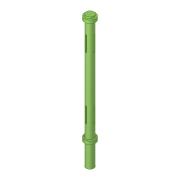
# Autodesk Inventor part: middleRod
Saved by Autodesk Inventor 2018 (Build 220112000, 112)
## iProperties
Created: 2017-11-16
Part Number: middleRod
Material: Aluminum 6061
Document SubType Name: Modeling
Designer: Udara Wanasinghe
Density: 2.7 g/cm^3
Appearance: Aluminum - Flat(1)
Mass: 41.1366 g
Surface Area: 69.3276 cm^2
Volume: 15.2358 cm^3
Author: Udara Wanasinghe
Autodesk Inventor part; units mm, degrees
ref_plane "XZ Plane" through (0, 0, 0) normal (0, 1, 0) x (-1, 0, 0)
ref_plane "XY Plane" through (0, 0, 0) normal (0, 0, 1) x (1, 0, 0)
sketch "Sketch1" plane through (0, 0, 0) normal (0, 1, 0) x (-1, 0, 0)
  circle A0 centre (0, 0) radius 5
  point P0 (0, 5)
  dimension "d0" = 10
  constraints: 1 coincident, 1 vertical alignment, 2 other
extrude "Extrusion1" add sketch "Sketch1" along normal blind 180
ref_plane "Work Plane1" through (-5, 0, 0) normal (1, 0, 0) x (0, 1, 0)
ref_plane "Work Plane4" through (0, 33, 0) normal (0, -1, 0) x (1, 0, 0)
sketch "Sketch7" plane through (0, 33, 0) normal (0, -1, 0) x (1, 0, 0)
  circle A0 centre (0, 0) radius 7
  dimension "d29" = 14
  constraints: 1 centre point, 1 coincident
  measures "d29" diameter of A0
extrude "Extrusion7" add sketch "Sketch7" along normal blind 4
ref_plane "Work Plane5" through (0, 165, 0) normal (0, 1, 0) x (1, 0, 0)
sketch "Sketch8" plane through (0, 165, 0) normal (0, 1, 0) x (1, 0, 0)
  circle A0 centre (0, 0) radius 7
  dimension "d33" = 14
  constraints: 1 centre point, 1 coincident
  measures "d33" diameter of A0
extrude "Extrusion8" add sketch "Sketch8" along normal blind 4
sketch "Sketch2" plane through (-5, 0, 0) normal (1, 0, 0) x (0, 1, 0)
  line L0 (150, -1) -> (130, -1)
  line L1 (130, -1) -> (130, 1)
  line L2 (130, 1) -> (150, 1)
  line L3 (150, 1) -> (150, -1)
  line L4 (150, 0) -> (130, 0) construction
  line L5 (180, -5) -> (180, 5) construction
  line L6 (180, 0) -> (0, 0) construction
  line L7 (0, 5) -> (0, -5) construction
  line L8 (70, -1) -> (50, -1)
  line L9 (50, -1) -> (50, 1)
  line L10 (50, 1) -> (70, 1)
  line L11 (70, 1) -> (70, -1)
  line L12 (70, 0) -> (50, 0) construction
  line L13 (165, 7) -> (165, -7) projected
  line L14 (33, -7) -> (33, 7) projected
  line L15 (169, -7) -> (169, 7) projected
  dimension "d3" = 20
  dimension "d4" = 2
  dimension "d6" = 20
  dimension "d7" = 2
  dimension "d36" = 15
  dimension "d37" = 17
  dimension "d38" = 60
  dimension "d40" = 15
  dimension "d41" = 33
  constraints: 22 end point, 5 midpoint, 4 parallel, 3 perpendicular, 2 collinear, 2 horizontal
  measures "d3" distance of L1.end L2.end
  measures "d4" distance of L0.end L1.end
  measures "d6" distance of L9.end L10.end
  measures "d7" distance of L8.end L9.end
  measures "d36" distance between parallel lines of L13 L3
  measures "d37" distance between parallel lines of L14 L9
  measures "d38" distance between parallel lines of L11 L1
  measures "d40" distance between parallel lines of L5 L13
  measures "d41" distance between parallel lines of L14 L7
extrude "Extrusion2" cut sketch "Sketch2" along normal blind 2
pattern_circular "Circular Pattern1" count 4 over 360 about axis through (0, -10, 0) along (0, 1, 0) of "Extrusion2"
sketch "Sketch9" plane through (0, 180, 0) normal (0, 1, 0) x (1, 0, 0)
  circle A0 centre (0, 0) radius 5
  dimension "d42" = 10
  constraints: 1 centre point, 1 coincident
  measures "d42" diameter of A0
extrude "Extrusion9" cut sketch "Sketch9" against normal blind 9
body "Solid1"
